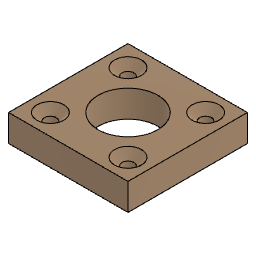
X platform support top (Autodesk Fusion 360 design; units mm, degrees)
Autodesk Fusion 360 part; units mm, degrees
sketch "Sketch1" plane through (0, 0, 0) normal (0, 0, 1) x (1, 0, 0)
  line L0 (20, 20) -> (-20, 20)
  line L1 (-20, 20) -> (-20, -20)
  line L2 (-20, -20) -> (20, -20)
  line L3 (20, -20) -> (20, 20)
  line L4 (20, 20) -> (-20, -20) construction
  line L5 (-20, 20) -> (20, -20) construction
  circle A0 centre (0, 0) radius 10
  line L6 (13, -13) -> (-13, -13) construction
  line L7 (-13, -13) -> (-13, 13) construction
  line L8 (-13, 13) -> (13, 13) construction
  line L9 (13, 13) -> (13, -13) construction
  line L10 (13, -13) -> (-13, 13) construction
  line L11 (-13, -13) -> (13, 13) construction
  circle A1 centre (-13, 13) radius 2
  circle A2 centre (13, 13) radius 2
  circle A3 centre (13, -13) radius 2
  circle A4 centre (-13, -13) radius 2
  dimension "d1" = 40
  dimension "d2" = 40
  dimension "d3" = 20
  dimension "d6" = 26
  dimension "d7" = 26
  dimension "d8" = 4
  dimension "d9" = 4
  dimension "d10" = 4
  dimension "d11" = 4
  constraint perpendicular L0 L1
  constraint parallel L0 L2
  constraint parallel L1 L3
  constraint horizontal L0
  constraint coincident L4 A0.centre
  constraint coincident L5 A0.centre
  constraint coincident A0.centre origin
  constraint perpendicular L6 L7
  constraint parallel L6 L8
  constraint parallel L7 L9
  constraint horizontal L6
  constraint coincident L10 A0.centre
  constraint coincident L11 A0.centre
  constraint coincident L7.end L8.start
  constraint coincident L8.end L9.start
  constraint coincident L6.start L9.end
  constraint coincident L6.end L7.start
  measures "d1" distance of L1.end L2.end
  measures "d2" distance of L0.end L1.end
  measures "d3" diameter of A0
  measures "d6" distance of L7.end L8.end
  measures "d7" distance of L6.end L7.end L0.start
  measures "d8" diameter of A1
  measures "d9" diameter of A2
  measures "d10" diameter of A3
  measures "d11" diameter of A4
extrude "Extrude1" add sketch "Sketch1" along normal blind 9
chamfer "Chamfer1" distance 2.5 angle 45 4 edges at (-14.8647, 13.7232, 9) (-14.8647, -12.2768, 9) (11.1353, -12.2768, 9) (11.1353, 13.7232, 9)
equation "d9 = d8"
equation "d10 = d8"
equation "d11 = d8"
named bodies: "Support top"
